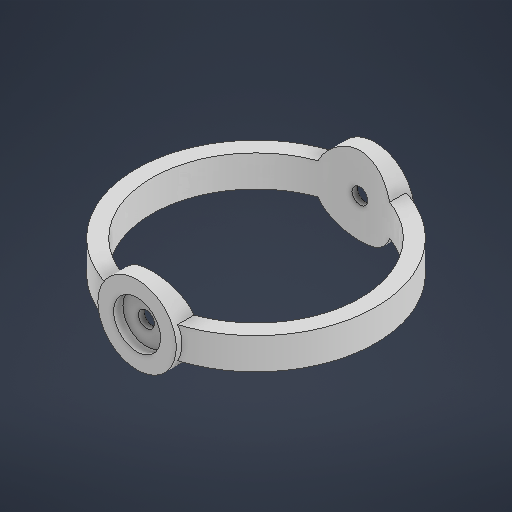
# Autodesk Inventor part: tubeHolder
Saved by Autodesk Inventor 2025.2 (Build 292293000, 293)
## iProperties
Created: 2025-02-28
Part Number: tubeHolder
Material: Generic
Document SubType Name: Modeling
Designer: huj31
Density: 1 g/cm^3
Appearance: Default
Author: huj31
Autodesk Inventor part; units mm, degrees
ref_plane "YZ Plane" through (0, 0, 0) normal (1, 0, 0) x (0, 1, 0)
ref_plane "XZ Plane" through (0, 0, 0) normal (0, 1, 0) x (-1, 0, 0)
ref_plane "XY Plane" through (0, 0, 0) normal (0, 0, 1) x (1, 0, 0)
sketch "Sketch1" plane through (0, 0, 0) normal (0, 1, 0) x (-1, 0, 0)
  circle A0 centre (0, 0) radius 33.25
  circle A1 centre (0, 0) radius 38.25
  dimension "d0" = 66.5
  dimension "d1" = 76.5
  constraints: 2 centre point, 2 coincident
  measures "d0" diameter of A0
  measures "d1" diameter of A1
extrude "Extrusion1" add sketch "Sketch1" along normal mid plane 10
sketch "Sketch2" plane through (0, 0, 0) normal (0, 0, 1) x (1, 0, 0)
  circle A0 centre (0, 0) radius 7.5
  circle A1 centre (0, 0) radius 12.5
  circle A2 centre (0, 0) radius 2.5
  dimension "d4" = 15
  dimension "d5" = 25
  dimension "d12" = 5
  constraints: 3 centre point, 3 coincident
  measures "d4" diameter of A0
  measures "d5" diameter of A1
  measures "d12" diameter of A2
extrude "Extrusion2" add sketch "Sketch2" along normal mid plane 76 contours A1
extrude "Extrusion3" cut sketch "Sketch2" along normal mid plane 79 contours A0 | A2
extrude "Extrusion4" add sketch "Sketch2" along normal mid plane 70 contours A0 | A2
extrude "Extrusion5" cut sketch "Sketch2" along normal mid plane 70 contours A2
extrude "Extrusion6" cut sketch "Sketch1" along normal mid plane 70 contours A0
body "Solid1"
